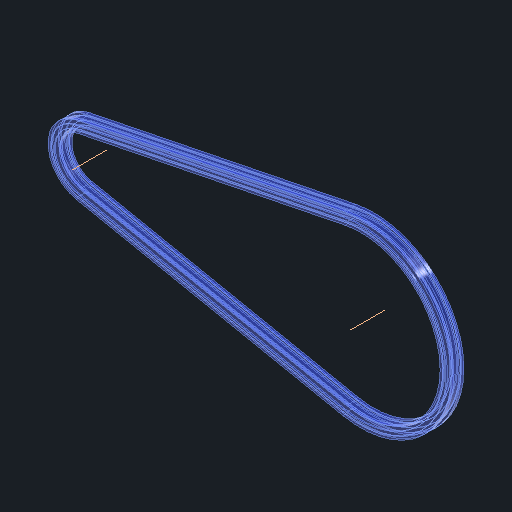
# Autodesk Inventor part: Roller Chain
Saved by Autodesk Inventor 2027 (Build 310192000, 192)
## iProperties
CustomPartVersion: 1
Created: 2026-06-06
Part Number: Roller Chain
Material: Generic
Document SubType Name: Modeling
Designer: W Ahmad
Density: 1 g/cm^3
Appearance: Clear - Blue
Author: W Ahmad
Autodesk Inventor part; units mm, degrees
ref_plane "Work Plane2" through (-254.3605, 0, 0) normal (-1, 0, 0) x (0, 0, 1)
ref_plane "Work Plane3" through (127, 0, 0) normal (-0.9976688, -0.0682424, 0) x (0, 0, 1)
sketch "Path" plane through (0, 0, 0) normal (0, 0, 1) x (1, 0, 0)
  arc A0 (-262.429, 39.8782) -> (-262.429, -39.8782) centre (-254.3605, 0) ccw
  arc A1 (103.9341, -114.0033) -> (103.9341, 114.0033) centre (127, 0) ccw
  line L0 (103.9341, -114.0033) -> (-262.429, -39.8782)
  line L1 (-262.429, 39.8782) -> (103.9341, 114.0033)
  dimension "d31" = 15.0114
  constraints: 4 end point, 4 point on circle, 2 centre point
ref_plane "Section Plane" through (-262.429, -39.8782, 0) normal (0.9801397, -0.1983084, 0) x (0, 0, 1)
sketch "Section Sketch" plane through (-262.429, -39.8782, 0) normal (0.9801397, -0.1983084, 0) x (0, 0, 1)
  line L0 (-10.541, -2.54) -> (10.541, -2.54)
  line L1 (10.541, -2.54) -> (10.541, 2.54)
  line L2 (10.541, 2.54) -> (-10.541, 2.54)
  line L3 (-10.541, 2.54) -> (-10.541, -2.54)
  line L4 (-4.7625, -5.08) -> (4.7625, -5.08)
  line L5 (4.7625, -5.08) -> (4.7625, 5.08)
  line L6 (4.7625, 5.08) -> (-4.7625, 5.08)
  line L7 (-4.7625, 5.08) -> (-4.7625, -5.08)
  line L8 (-4.7625, 0) -> (4.7625, 0) construction
  line L9 (-8.8265, -7.5057) -> (-4.7625, -7.5057)
  line L10 (-4.7625, -7.5057) -> (-4.7625, 7.5057)
  line L11 (-4.7625, 7.5057) -> (-8.8265, 7.5057)
  line L12 (-8.8265, 7.5057) -> (-8.8265, -7.5057)
  line L13 (4.7625, -7.5057) -> (8.8265, -7.5057)
  line L14 (8.8265, -7.5057) -> (8.8265, 7.5057)
  line L15 (8.8265, 7.5057) -> (4.7625, 7.5057)
  line L16 (4.7625, 7.5057) -> (4.7625, -7.5057)
  line L17 (-10.541, 0) -> (10.541, 0) construction
  point P0 (0, 0)
  point P1 (0, 0)
  dimension "d21" = 5.08
  dimension "d22" = 10.16
  dimension "d23" = 9.525
  dimension "d24" = 4.064
  dimension "d31" = 15.0114
  dimension "d32" = 21.082
  constraints: 36 end point, 8 midpoint, 8 parallel, 4 horizontal, 4 perpendicular, 3 collinear, 1 coincident, 1 other
  measures "d21" distance between parallel lines of L2 L0
  measures "d22" distance between parallel lines of L6 L4
  measures "d23" distance between parallel lines of L5 L7
  measures "d24" distance between parallel lines of L12 L10
  measures "d31" distance between parallel lines of L11 L9
  measures "d32" distance between parallel lines of L1 L3
sweep "Solid" add profiles "Section Sketch" path "Path"
pattern_of_one "Strand Pattern"
equation "\"d21\" = da_d2"
equation "\"d22\" = da_d1"
equation "\"d23\" = da_b1"
equation "\"d24\" = da_t1 + da_t2"
equation "\"d30\" = da_pt"
equation "\"da_p\" = 15.875"
equation "\"da_b1\" = 9.525"
equation "\"da_h2\" = 15.0114"
equation "\"da_h3\" = 13.0048"
equation "\"da_d1\" = 10.16"
equation "\"da_d2\" = 5.08"
equation "\"da_pt\" = 18.1102"
equation "\"da_b\" = 21.082"
equation "\"da_t1\" = 2.032"
equation "\"da_t2\" = 2.032"
body "Solid1"
